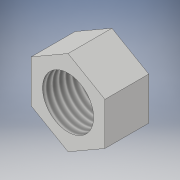
# Autodesk Inventor part: .875nut
Saved by Autodesk Inventor 2017 (Build 210142000, 142)
## iProperties
Created: 2017-04-26
Part Number: .875nut
Material: Generic
Document SubType Name: Modeling
Designer: User
Density: 1 g/cm^3
Appearance: Default
Author: User
Autodesk Inventor part; units mm, degrees
ref_plane "YZ Plane" through (0, 0, 0) normal (1, 0, 0) x (0, 1, 0)
ref_plane "XZ Plane" through (0, 0, 0) normal (0, 1, 0) x (-1, 0, 0)
ref_plane "XY Plane" through (0, 0, 0) normal (0, 0, 1) x (1, 0, 0)
sketch "Sketch1" plane through (0, 0, 0) normal (0, 0, 1) x (1, 0, 0)
  circle A0 centre (0, 0) radius 11.1125
  line L0 (0, 18.4776) -> (16.0021, 9.2388)
  line L1 (16.0021, 9.2388) -> (16.0021, -9.2388)
  line L2 (16.0021, -9.2388) -> (0, -18.4776)
  line L3 (0, -18.4776) -> (-16.0021, -9.2388)
  line L4 (-16.0021, -9.2388) -> (-16.0021, 9.2388)
  line L5 (-16.0021, 9.2388) -> (0, 18.4776)
  dimension "d0" = 22.225
  constraints: 12 end point, 2 coincident, 1 centre point, 13 other
  measures "d0" diameter of A0
extrude "Extrusion1" add sketch "Sketch1" along normal blind 19.05
thread "Thread1" size "7/8-9 UNC" class "2B" standard "ANSI Unified Screw Threads" full length
body "Solid1"
